Autodesk Fusion 360 part; units mm, degrees
(part 2 of 3)
  spline S19 degree 5 poles (-84.2227, 13.9647) (-84.2245, 13.9707) (-84.2281, 13.9827) (-84.2336, 14.0007) (-84.2409, 14.0246) (-84.2503, 14.0545) (-84.2597, 14.0843) (-84.2693, 14.114) (-84.279, 14.1436) (-84.2888, 14.1731) (-84.2987, 14.2026) (-84.3088, 14.2319) (-84.3189, 14.2612) (-84.3292, 14.2903) (-84.3396, 14.3194) (-84.3502, 14.3484) (-84.3608, 14.3773) (-84.3716, 14.4061) (-84.3825, 14.4348) (-84.3935, 14.4635) (-84.4046, 14.492) (-84.4159, 14.5204) (-84.4273, 14.5488) (-84.4388, 14.577) (-84.4504, 14.6051) (-84.4622, 14.6332) (-84.4741, 14.6611) (-84.4861, 14.6889) (-84.4982, 14.7166) (-84.5105, 14.7442) (-84.5229, 14.7718) (-84.5354, 14.7992) (-84.5481, 14.8264) (-84.5609, 14.8536) (-84.5738, 14.8807) (-84.5869, 14.9076) (-84.6, 14.9345) (-84.6134, 14.9612) (-84.6268, 14.9878) (-84.6404, 15.0143) (-84.6542, 15.0406) (-84.668, 15.0668) (-84.6821, 15.0929) (-84.6962, 15.1189) (-84.7105, 15.1447) (-84.725, 15.1704) (-84.7396, 15.196) (-84.7543, 15.2214) (-84.7692, 15.2467) (-84.7842, 15.2719) (-84.7994, 15.2969) (-84.8148, 15.3217) (-84.8303, 15.3464) (-84.846, 15.3709) (-84.8619, 15.3952) (-84.878, 15.4194) (-84.8941, 15.4435) (-84.9105, 15.4674) (-84.927, 15.4911) (-84.9436, 15.5146) (-84.9605, 15.5379) (-84.9777, 15.561) (-84.9951, 15.5838) (-85.0128, 15.6063) (-85.0307, 15.6286) (-85.0488, 15.6506) (-85.067, 15.6726) (-85.0853, 15.6944) (-85.1038, 15.716) (-85.1226, 15.7372) (-85.142, 15.7579) (-85.1581, 15.7737) (-85.1706, 15.7852) (-85.1791, 15.7926) (-85.1834, 15.7963) knots -1 -1 -1 -1 -1 -1 -0.98571429 -0.97142857 -0.95714286 -0.94285714 -0.92857143 -0.91428571 -0.9 -0.88571429 -0.87142857 -0.85714286 -0.84285714 -0.82857143 -0.81428571 -0.8 -0.78571429 -0.77142857 -0.75714286 -0.74285714 -0.72857143 -0.71428571 -0.7 -0.68571429 -0.67142857 -0.65714286 -0.64285714 -0.62857143 -0.61428571 -0.6 -0.58571429 -0.57142857 -0.55714286 -0.54285714 -0.52857143 -0.51428571 -0.5 -0.48571429 -0.47142857 -0.45714286 -0.44285714 -0.42857143 -0.41428571 -0.4 -0.38571429 -0.37142857 -0.35714286 -0.34285714 -0.32857143 -0.31428571 -0.3 -0.28571429 -0.27142857 -0.25714286 -0.24285714 -0.22857143 -0.21428571 -0.2 -0.18571429 -0.17142857 -0.15714286 -0.14285714 -0.12857143 -0.11428571 -0.1 -0.08571429 -0.07142857 -0.05714286 -0.04285714 -0.02857143 -0.01428571 0 0 0 0 0 0
  line L19 (-85.1834, 15.7963) -> (-85.554, 16.1126)
  arc A39 (-85.5658, 16.2528) -> (-85.554, 16.1126) centre (-85.4891, 16.1886) ccw
  arc A40 (-85.5658, 16.2528) -> (-84.943, 17.0645) centre (-94.8448, 24.0176) ccw
  arc A41 (-84.8044, 17.0894) -> (-84.943, 17.0645) centre (-84.8611, 17.0071) ccw
  line L20 (-84.8044, 17.0894) -> (-84.4031, 16.8133)
  spline S20 degree 5 poles (-84.4031, 16.8133) (-84.3984, 16.8101) (-84.389, 16.8038) (-84.3747, 16.7947) (-84.3552, 16.7833) (-84.3302, 16.7699) (-84.3049, 16.7572) (-84.2792, 16.7449) (-84.2534, 16.7328) (-84.2275, 16.7209) (-84.2015, 16.7092) (-84.1753, 16.6977) (-84.149, 16.6864) (-84.1225, 16.6755) (-84.0958, 16.6649) (-84.0689, 16.6546) (-84.0418, 16.6446) (-84.0147, 16.6348) (-83.9874, 16.6252) (-83.96, 16.6158) (-83.9324, 16.6066) (-83.9048, 16.5975) (-83.8771, 16.5887) (-83.8492, 16.5801) (-83.8213, 16.5717) (-83.7932, 16.5634) (-83.765, 16.5554) (-83.7367, 16.5476) (-83.7083, 16.5399) (-83.6798, 16.5325) (-83.6513, 16.5252) (-83.6226, 16.518) (-83.5939, 16.5111) (-83.565, 16.5043) (-83.5361, 16.4977) (-83.5071, 16.4912) (-83.478, 16.4849) (-83.4488, 16.4788) (-83.4196, 16.4729) (-83.3903, 16.4671) (-83.3608, 16.4614) (-83.3314, 16.456) (-83.3018, 16.4506) (-83.2722, 16.4455) (-83.2425, 16.4405) (-83.2127, 16.4356) (-83.1828, 16.4309) (-83.1529, 16.4263) (-83.1229, 16.4219) (-83.0929, 16.4177) (-83.0627, 16.4136) (-83.0326, 16.4096) (-83.0023, 16.4058) (-82.972, 16.4021) (-82.9416, 16.3986) (-82.9112, 16.3952) (-82.8807, 16.392) (-82.8501, 16.3889) (-82.8195, 16.386) (-82.7888, 16.3832) (-82.7581, 16.3805) (-82.7273, 16.378) (-82.6965, 16.3756) (-82.6656, 16.3734) (-82.6346, 16.3712) (-82.6036, 16.3693) (-82.5726, 16.3674) (-82.5415, 16.3657) (-82.5103, 16.3642) (-82.4791, 16.3628) (-82.4478, 16.3615) (-82.4228, 16.3606) (-82.404, 16.3599) (-82.3914, 16.3595) (-82.3851, 16.3593) knots 0 0 0 0 0 0 0.01428571 0.02857143 0.04285714 0.05714286 0.07142857 0.08571429 0.1 0.11428571 0.12857143 0.14285714 0.15714286 0.17142857 0.18571429 0.2 0.21428571 0.22857143 0.24285714 0.25714286 0.27142857 0.28571429 0.3 0.31428571 0.32857143 0.34285714 0.35714286 0.37142857 0.38571429 0.4 0.41428571 0.42857143 0.44285714 0.45714286 0.47142857 0.48571429 0.5 0.51428571 0.52857143 0.54285714 0.55714286 0.57142857 0.58571429 0.6 0.61428571 0.62857143 0.64285714 0.65714286 0.67142857 0.68571429 0.7 0.71428571 0.72857143 0.74285714 0.75714286 0.77142857 0.78571429 0.8 0.81428571 0.82857143 0.84285714 0.85714286 0.87142857 0.88571429 0.9 0.91428571 0.92857143 0.94285714 0.95714286 0.97142857 0.98571429 1 1 1 1 1 1
  arc A42 (-82.3851, 16.3593) -> (-81.9827, 17.0564) centre (-94.8448, 24.0176) ccw
  spline S21 degree 5 poles (-81.9827, 17.0564) (-81.986, 17.0617) (-81.9926, 17.0724) (-82.0026, 17.0884) (-82.0159, 17.1096) (-82.0326, 17.136) (-82.0495, 17.1624) (-82.0664, 17.1886) (-82.0834, 17.2147) (-82.1005, 17.2406) (-82.1178, 17.2665) (-82.1351, 17.2923) (-82.1524, 17.3179) (-82.1699, 17.3434) (-82.1875, 17.3688) (-82.2052, 17.3941) (-82.223, 17.4193) (-82.2408, 17.4443) (-82.2588, 17.4692) (-82.2768, 17.494) (-82.295, 17.5187) (-82.3132, 17.5432) (-82.3315, 17.5676) (-82.3499, 17.5919) (-82.3685, 17.6161) (-82.3871, 17.6401) (-82.4058, 17.664) (-82.4246, 17.6878) (-82.4435, 17.7114) (-82.4625, 17.7349) (-82.4816, 17.7583) (-82.5008, 17.7815) (-82.5201, 17.8046) (-82.5395, 17.8275) (-82.559, 17.8503) (-82.5785, 17.873) (-82.5982, 17.8955) (-82.618, 17.9178) (-82.6379, 17.9401) (-82.6579, 17.9621) (-82.678, 17.984) (-82.6982, 18.0058) (-82.7185, 18.0273) (-82.7389, 18.0487) (-82.7594, 18.07) (-82.78, 18.0911) (-82.8007, 18.112) (-82.8215, 18.1328) (-82.8424, 18.1533) (-82.8635, 18.1737) (-82.8846, 18.194) (-82.9059, 18.214) (-82.9273, 18.2338) (-82.9488, 18.2534) (-82.9704, 18.2728) (-82.9922, 18.292) (-83.014, 18.311) (-83.036, 18.3299) (-83.0581, 18.3485) (-83.0803, 18.3669) (-83.1026, 18.3851) (-83.1252, 18.4029) (-83.1479, 18.4204) (-83.1708, 18.4376) (-83.1939, 18.4545) (-83.217, 18.4711) (-83.2403, 18.4876) (-83.2636, 18.5039) (-83.2871, 18.52) (-83.3108, 18.5356) (-83.3349, 18.5505) (-83.3545, 18.5617) (-83.3695, 18.5696) (-83.3797, 18.5746) (-83.3848, 18.577) knots -1 -1 -1 -1 -1 -1 -0.98571429 -0.97142857 -0.95714286 -0.94285714 -0.92857143 -0.91428571 -0.9 -0.88571429 -0.87142857 -0.85714286 -0.84285714 -0.82857143 -0.81428571 -0.8 -0.78571429 -0.77142857 -0.75714286 -0.74285714 -0.72857143 -0.71428571 -0.7 -0.68571429 -0.67142857 -0.65714286 -0.64285714 -0.62857143 -0.61428571 -0.6 -0.58571429 -0.57142857 -0.55714286 -0.54285714 -0.52857143 -0.51428571 -0.5 -0.48571429 -0.47142857 -0.45714286 -0.44285714 -0.42857143 -0.41428571 -0.4 -0.38571429 -0.37142857 -0.35714286 -0.34285714 -0.32857143 -0.31428571 -0.3 -0.28571429 -0.27142857 -0.25714286 -0.24285714 -0.22857143 -0.21428571 -0.2 -0.18571429 -0.17142857 -0.15714286 -0.14285714 -0.12857143 -0.11428571 -0.1 -0.08571429 -0.07142857 -0.05714286 -0.04285714 -0.02857143 -0.01428571 0 0 0 0 0 0
  line L21 (-83.3848, 18.577) -> (-83.8246, 18.7865)
  arc A43 (-83.8723, 18.9189) -> (-83.8246, 18.7865) centre (-83.7816, 18.8768) ccw
  arc A44 (-83.8723, 18.9189) -> (-83.4808, 19.8642) centre (-94.8448, 24.0176) ccw
  arc A45 (-83.3534, 19.9241) -> (-83.4808, 19.8642) centre (-83.3868, 19.8299) ccw
  line L22 (-83.3534, 19.9241) -> (-82.8942, 19.7613)
  spline S22 degree 5 poles (-82.8942, 19.7613) (-82.8889, 19.7594) (-82.8782, 19.7557) (-82.862, 19.7507) (-82.8402, 19.7447) (-82.8127, 19.7382) (-82.7849, 19.7325) (-82.7569, 19.7273) (-82.7289, 19.7223) (-82.7008, 19.7175) (-82.6726, 19.7129) (-82.6444, 19.7085) (-82.616, 19.7045) (-82.5876, 19.7008) (-82.559, 19.6975) (-82.5304, 19.6945) (-82.5017, 19.6918) (-82.4729, 19.6894) (-82.444, 19.6872) (-82.4151, 19.6852) (-82.3862, 19.6834) (-82.3571, 19.6818) (-82.3281, 19.6805) (-82.2989, 19.6793) (-82.2697, 19.6785) (-82.2405, 19.6778) (-82.2112, 19.6774) (-82.1818, 19.6771) (-82.1524, 19.6771) (-82.123, 19.6772) (-82.0935, 19.6775) (-82.064, 19.6781) (-82.0344, 19.6788) (-82.0048, 19.6797) (-81.9751, 19.6808) (-81.9455, 19.6821) (-81.9157, 19.6835) (-81.886, 19.6852) (-81.8562, 19.687) (-81.8263, 19.689) (-81.7965, 19.6912) (-81.7666, 19.6935) (-81.7366, 19.696) (-81.7067, 19.6987) (-81.6767, 19.7015) (-81.6467, 19.7046) (-81.6166, 19.7077) (-81.5865, 19.7111) (-81.5564, 19.7146) (-81.5263, 19.7183) (-81.4961, 19.7221) (-81.466, 19.7261) (-81.4358, 19.7302) (-81.4055, 19.7345) (-81.3753, 19.739) (-81.345, 19.7436) (-81.3147, 19.7484) (-81.2844, 19.7533) (-81.2541, 19.7584) (-81.2237, 19.7636) (-81.1933, 19.769) (-81.1629, 19.7745) (-81.1325, 19.7802) (-81.1021, 19.786) (-81.0717, 19.792) (-81.0412, 19.7981) (-81.0107, 19.8044) (-80.9802, 19.8108) (-80.9497, 19.8174) (-80.9192, 19.8241) (-80.8887, 19.8309) (-80.8643, 19.8365) (-80.8459, 19.8408) (-80.8337, 19.8436) (-80.8276, 19.8451) knots 0 0 0 0 0 0 0.01428571 0.02857143 0.04285714 0.05714286 0.07142857 0.08571429 0.1 0.11428571 0.12857143 0.14285714 0.15714286 0.17142857 0.18571429 0.2 0.21428571 0.22857143 0.24285714 0.25714286 0.27142857 0.28571429 0.3 0.31428571 0.32857143 0.34285714 0.35714286 0.37142857 0.38571429 0.4 0.41428571 0.42857143 0.44285714 0.45714286 0.47142857 0.48571429 0.5 0.51428571 0.52857143 0.54285714 0.55714286 0.57142857 0.58571429 0.6 0.61428571 0.62857143 0.64285714 0.65714286 0.67142857 0.68571429 0.7 0.71428571 0.72857143 0.74285714 0.75714286 0.77142857 0.78571429 0.8 0.81428571 0.82857143 0.84285714 0.85714286 0.87142857 0.88571429 0.9 0.91428571 0.92857143 0.94285714 0.95714286 0.97142857 0.98571429 1 1 1 1 1 1
  arc A46 (-80.8276, 19.8451) -> (-80.6193, 20.6225) centre (-94.8448, 24.0176) ccw
  spline S23 degree 5 poles (-80.6193, 20.6225) (-80.6238, 20.6268) (-80.633, 20.6354) (-80.6467, 20.6483) (-80.6651, 20.6654) (-80.6881, 20.6865) (-80.7112, 20.7076) (-80.7343, 20.7285) (-80.7575, 20.7493) (-80.7808, 20.77) (-80.8041, 20.7905) (-80.8275, 20.8109) (-80.8509, 20.8312) (-80.8744, 20.8513) (-80.898, 20.8713) (-80.9216, 20.8911) (-80.9453, 20.9108) (-80.969, 20.9304) (-80.9928, 20.9498) (-81.0166, 20.9691) (-81.0405, 20.9882) (-81.0645, 21.0072) (-81.0885, 21.0261) (-81.1126, 21.0448) (-81.1368, 21.0633) (-81.161, 21.0817) (-81.1852, 21.1) (-81.2095, 21.118) (-81.2339, 21.136) (-81.2583, 21.1538) (-81.2828, 21.1714) (-81.3074, 21.1889) (-81.332, 21.2062) (-81.3567, 21.2233) (-81.3814, 21.2403) (-81.4062, 21.2571) (-81.431, 21.2737) (-81.4559, 21.2902) (-81.4809, 21.3065) (-81.5059, 21.3226) (-81.5309, 21.3386) (-81.5561, 21.3544) (-81.5813, 21.37) (-81.6065, 21.3854) (-81.6318, 21.4006) (-81.6572, 21.4156) (-81.6826, 21.4305) (-81.7081, 21.4451) (-81.7336, 21.4596) (-81.7592, 21.4738) (-81.7849, 21.4879) (-81.8106, 21.5017) (-81.8364, 21.5153) (-81.8623, 21.5287) (-81.8882, 21.5418) (-81.9142, 21.5548) (-81.9402, 21.5675) (-81.9663, 21.58) (-81.9924, 21.5923) (-82.0186, 21.6044) (-82.0449, 21.6161) (-82.0713, 21.6275) (-82.0978, 21.6385) (-82.1244, 21.6492) (-82.151, 21.6595) (-82.1777, 21.6696) (-82.2044, 21.6795) (-82.2312, 21.6892) (-82.258, 21.6987) (-82.285, 21.7076) (-82.3121, 21.7158) (-82.3339, 21.7215) (-82.3505, 21.7252) (-82.3616, 21.7274) (-82.3672, 21.7284) knots -1 -1 -1 -1 -1 -1 -0.98571429 -0.97142857 -0.95714286 -0.94285714 -0.92857143 -0.91428571 -0.9 -0.88571429 -0.87142857 -0.85714286 -0.84285714 -0.82857143 -0.81428571 -0.8 -0.78571429 -0.77142857 -0.75714286 -0.74285714 -0.72857143 -0.71428571 -0.7 -0.68571429 -0.67142857 -0.65714286 -0.64285714 -0.62857143 -0.61428571 -0.6 -0.58571429 -0.57142857 -0.55714286 -0.54285714 -0.52857143 -0.51428571 -0.5 -0.48571429 -0.47142857 -0.45714286 -0.44285714 -0.42857143 -0.41428571 -0.4 -0.38571429 -0.37142857 -0.35714286 -0.34285714 -0.32857143 -0.31428571 -0.3 -0.28571429 -0.27142857 -0.25714286 -0.24285714 -0.22857143 -0.21428571 -0.2 -0.18571429 -0.17142857 -0.15714286 -0.14285714 -0.12857143 -0.11428571 -0.1 -0.08571429 -0.07142857 -0.05714286 -0.04285714 -0.02857143 -0.01428571 0 0 0 0 0 0
  line L23 (-82.3672, 21.7284) -> (-82.8462, 21.817)
  arc A47 (-82.9266, 21.9326) -> (-82.8462, 21.817) centre (-82.8281, 21.9153) ccw
  arc A48 (-82.9266, 21.9326) -> (-82.793, 22.947) centre (-94.8448, 24.0176) ccw
  arc A49 (-82.6855, 23.0378) -> (-82.793, 22.947) centre (-82.6934, 22.9381) ccw
  line L24 (-82.6855, 23.0378) -> (-82.1998, 22.9993)
  spline S24 degree 5 poles (-82.1998, 22.9993) (-82.1942, 22.9989) (-82.1829, 22.9981) (-82.166, 22.9974) (-82.1434, 22.9973) (-82.1151, 22.9982) (-82.0867, 22.9998) (-82.0584, 23.002) (-82.03, 23.0045) (-82.0016, 23.0071) (-81.9732, 23.01) (-81.9448, 23.0131) (-81.9164, 23.0165) (-81.888, 23.0203) (-81.8595, 23.0244) (-81.8311, 23.029) (-81.8027, 23.0338) (-81.7742, 23.0389) (-81.7458, 23.0443) (-81.7173, 23.0498) (-81.6889, 23.0556) (-81.6605, 23.0616) (-81.632, 23.0678) (-81.6036, 23.0743) (-81.5752, 23.081) (-81.5467, 23.0879) (-81.5183, 23.0951) (-81.4899, 23.1024) (-81.4615, 23.11) (-81.4331, 23.1177) (-81.4047, 23.1257) (-81.3763, 23.1338) (-81.3479, 23.1422) (-81.3196, 23.1507) (-81.2912, 23.1595) (-81.2629, 23.1684) (-81.2345, 23.1775) (-81.2062, 23.1868) (-81.1779, 23.1962) (-81.1496, 23.2059) (-81.1213, 23.2157) (-81.093, 23.2257) (-81.0648, 23.2359) (-81.0365, 23.2462) (-81.0083, 23.2568) (-80.9801, 23.2674) (-80.9519, 23.2783) (-80.9237, 23.2893) (-80.8955, 23.3005) (-80.8674, 23.3118) (-80.8392, 23.3233) (-80.8111, 23.335) (-80.783, 23.3468) (-80.7549, 23.3588) (-80.7268, 23.3709) (-80.6988, 23.3832) (-80.6708, 23.3957) (-80.6428, 23.4083) (-80.6148, 23.421) (-80.5868, 23.4339) (-80.5589, 23.447) (-80.5309, 23.4602) (-80.503, 23.4736) (-80.4752, 23.4871) (-80.4473, 23.5007) (-80.4195, 23.5145) (-80.3917, 23.5285) (-80.3639, 23.5425) (-80.3361, 23.5568) (-80.3084, 23.5712) (-80.2806, 23.5857) (-80.2585, 23.5974) (-80.2419, 23.6062) (-80.2308, 23.6122) (-80.2253, 23.6152) knots 0 0 0 0 0 0 0.01428571 0.02857143 0.04285714 0.05714286 0.07142857 0.08571429 0.1 0.11428571 0.12857143 0.14285714 0.15714286 0.17142857 0.18571429 0.2 0.21428571 0.22857143 0.24285714 0.25714286 0.27142857 0.28571429 0.3 0.31428571 0.32857143 0.34285714 0.35714286 0.37142857 0.38571429 0.4 0.41428571 0.42857143 0.44285714 0.45714286 0.47142857 0.48571429 0.5 0.51428571 0.52857143 0.54285714 0.55714286 0.57142857 0.58571429 0.6 0.61428571 0.62857143 0.64285714 0.65714286 0.67142857 0.68571429 0.7 0.71428571 0.72857143 0.74285714 0.75714286 0.77142857 0.78571429 0.8 0.81428571 0.82857143 0.84285714 0.85714286 0.87142857 0.88571429 0.9 0.91428571 0.92857143 0.94285714 0.95714286 0.97142857 0.98571429 1 1 1 1 1 1
  arc A50 (-80.2253, 23.6152) -> (-80.2253, 24.42) centre (-94.8448, 24.0176) ccw
  spline S25 degree 5 poles (-80.2253, 24.42) (-80.2308, 24.423) (-80.2419, 24.429) (-80.2585, 24.4378) (-80.2806, 24.4495) (-80.3084, 24.4641) (-80.3361, 24.4784) (-80.3639, 24.4927) (-80.3917, 24.5067) (-80.4195, 24.5207) (-80.4473, 24.5345) (-80.4752, 24.5481) (-80.503, 24.5616) (-80.5309, 24.575) (-80.5589, 24.5882) (-80.5868, 24.6013) (-80.6148, 24.6142) (-80.6428, 24.6269) (-80.6708, 24.6395) (-80.6988, 24.652) (-80.7268, 24.6643) (-80.7549, 24.6764) (-80.783, 24.6884) (-80.8111, 24.7002) (-80.8392, 24.7119) (-80.8674, 24.7234) (-80.8955, 24.7347) (-80.9237, 24.7459) (-80.9519, 24.7569) (-80.9801, 24.7678) (-81.0083, 24.7785) (-81.0365, 24.789) (-81.0648, 24.7993) (-81.093, 24.8095) (-81.1213, 24.8195) (-81.1496, 24.8293) (-81.1779, 24.839) (-81.2062, 24.8484) (-81.2345, 24.8577) (-81.2629, 24.8668) (-81.2912, 24.8757) (-81.3196, 24.8845) (-81.3479, 24.893) (-81.3763, 24.9014) (-81.4047, 24.9095) (-81.4331, 24.9175) (-81.4615, 24.9252) (-81.4899, 24.9328) (-81.5183, 24.9402) (-81.5467, 24.9473) (-81.5752, 24.9542) (-81.6036, 24.9609) (-81.632, 24.9674) (-81.6605, 24.9736) (-81.6889, 24.9796) (-81.7173, 24.9854) (-81.7458, 24.9909) (-81.7742, 24.9963) (-81.8027, 25.0014) (-81.8311, 25.0062) (-81.8595, 25.0108) (-81.888, 25.0149) (-81.9164, 25.0187) (-81.9448, 25.0221) (-81.9732, 25.0252) (-82.0016, 25.0281) (-82.03, 25.0307) (-82.0584, 25.0332) (-82.0867, 25.0354) (-82.1151, 25.0371) (-82.1434, 25.0379) (-82.166, 25.0378) (-82.1829, 25.0371) (-82.1942, 25.0363) (-82.1998, 25.0359) knots -1 -1 -1 -1 -1 -1 -0.98571429 -0.97142857 -0.95714286 -0.94285714 -0.92857143 -0.91428571 -0.9 -0.88571429 -0.87142857 -0.85714286 -0.84285714 -0.82857143 -0.81428571 -0.8 -0.78571429 -0.77142857 -0.75714286 -0.74285714 -0.72857143 -0.71428571 -0.7 -0.68571429 -0.67142857 -0.65714286 -0.64285714 -0.62857143 -0.61428571 -0.6 -0.58571429 -0.57142857 -0.55714286 -0.54285714 -0.52857143 -0.51428571 -0.5 -0.48571429 -0.47142857 -0.45714286 -0.44285714 -0.42857143 -0.41428571 -0.4 -0.38571429 -0.37142857 -0.35714286 -0.34285714 -0.32857143 -0.31428571 -0.3 -0.28571429 -0.27142857 -0.25714286 -0.24285714 -0.22857143 -0.21428571 -0.2 -0.18571429 -0.17142857 -0.15714286 -0.14285714 -0.12857143 -0.11428571 -0.1 -0.08571429 -0.07142857 -0.05714286 -0.04285714 -0.02857143 -0.01428571 0 0 0 0 0 0
  line L25 (-82.1998, 25.0359) -> (-82.6855, 24.9974)
  arc A51 (-82.793, 25.0883) -> (-82.6855, 24.9974) centre (-82.6934, 25.0971) ccw
  arc A52 (-82.793, 25.0883) -> (-82.9266, 26.1027) centre (-94.8448, 24.0176) ccw
  arc A53 (-82.8462, 26.2182) -> (-82.9266, 26.1027) centre (-82.8281, 26.1199) ccw
  line L26 (-82.8462, 26.2182) -> (-82.3672, 26.3068)
  spline S26 degree 5 poles (-82.3672, 26.3068) (-82.3616, 26.3078) (-82.3505, 26.31) (-82.3339, 26.3137) (-82.3121, 26.3194) (-82.285, 26.3276) (-82.258, 26.3365) (-82.2312, 26.346) (-82.2044, 26.3557) (-82.1777, 26.3656) (-82.151, 26.3757) (-82.1244, 26.386) (-82.0978, 26.3967) (-82.0713, 26.4077) (-82.0449, 26.4191) (-82.0186, 26.4309) (-81.9924, 26.4429) (-81.9663, 26.4552) (-81.9402, 26.4677) (-81.9142, 26.4804) (-81.8882, 26.4934) (-81.8623, 26.5065) (-81.8364, 26.5199) (-81.8106, 26.5335) (-81.7849, 26.5473) (-81.7592, 26.5614) (-81.7336, 26.5756) (-81.7081, 26.5901) (-81.6826, 26.6047) (-81.6572, 26.6196) (-81.6318, 26.6346) (-81.6065, 26.6498) (-81.5813, 26.6652) (-81.5561, 26.6808) (-81.5309, 26.6966) (-81.5059, 26.7126) (-81.4809, 26.7287) (-81.4559, 26.745) (-81.431, 26.7615) (-81.4062, 26.7781) (-81.3814, 26.7949) (-81.3567, 26.8119) (-81.332, 26.829) (-81.3074, 26.8464) (-81.2828, 26.8638) (-81.2583, 26.8814) (-81.2339, 26.8992) (-81.2095, 26.9172) (-81.1852, 26.9352) (-81.161, 26.9535) (-81.1368, 26.9719) (-81.1126, 26.9904) (-81.0885, 27.0091) (-81.0645, 27.028) (-81.0405, 27.047) (-81.0166, 27.0661) (-80.9928, 27.0854) (-80.969, 27.1048) (-80.9453, 27.1244) (-80.9216, 27.1441) (-80.898, 27.1639) (-80.8744, 27.1839) (-80.8509, 27.204) (-80.8275, 27.2243) (-80.8041, 27.2447) (-80.7808, 27.2652) (-80.7575, 27.2859) (-80.7343, 27.3067) (-80.7112, 27.3276) (-80.6881, 27.3487) (-80.6651, 27.3699) (-80.6467, 27.3869) (-80.633, 27.3998) (-80.6238, 27.4084) (-80.6193, 27.4127) knots 0 0 0 0 0 0 0.01428571 0.02857143 0.04285714 0.05714286 0.07142857 0.08571429 0.1 0.11428571 0.12857143 0.14285714 0.15714286 0.17142857 0.18571429 0.2 0.21428571 0.22857143 0.24285714 0.25714286 0.27142857 0.28571429 0.3 0.31428571 0.32857143 0.34285714 0.35714286 0.37142857 0.38571429 0.4 0.41428571 0.42857143 0.44285714 0.45714286 0.47142857 0.48571429 0.5 0.51428571 0.52857143 0.54285714 0.55714286 0.57142857 0.58571429 0.6 0.61428571 0.62857143 0.64285714 0.65714286 0.67142857 0.68571429 0.7 0.71428571 0.72857143 0.74285714 0.75714286 0.77142857 0.78571429 0.8 0.81428571 0.82857143 0.84285714 0.85714286 0.87142857 0.88571429 0.9 0.91428571 0.92857143 0.94285714 0.95714286 0.97142857 0.98571429 1 1 1 1 1 1
  arc A54 (-80.6193, 27.4127) -> (-80.8276, 28.1901) centre (-94.8448, 24.0176) ccw
  spline S27 degree 5 poles (-80.8276, 28.1901) (-80.8337, 28.1916) (-80.8459, 28.1944) (-80.8643, 28.1987) (-80.8887, 28.2043) (-80.9192, 28.2111) (-80.9497, 28.2178) (-80.9802, 28.2244) (-81.0107, 28.2308) (-81.0412, 28.2371) (-81.0717, 28.2432) (-81.1021, 28.2492) (-81.1325, 28.255) (-81.1629, 28.2607) (-81.1933, 28.2662) (-81.2237, 28.2716) (-81.2541, 28.2768) (-81.2844, 28.2819) (-81.3147, 28.2868) (-81.345, 28.2916) (-81.3753, 28.2962) (-81.4055, 28.3007) (-81.4358, 28.305) (-81.466, 28.3091) (-81.4961, 28.3131) (-81.5263, 28.3169) (-81.5564, 28.3206) (-81.5865, 28.3241) (-81.6166, 28.3275) (-81.6467, 28.3307) (-81.6767, 28.3337) (-81.7067, 28.3365) (-81.7366, 28.3392) (-81.7666, 28.3417) (-81.7965, 28.3441) (-81.8263, 28.3462) (-81.8562, 28.3482) (-81.886, 28.35) (-81.9157, 28.3517) (-81.9455, 28.3531) (-81.9751, 28.3544) (-82.0048, 28.3555) (-82.0344, 28.3564) (-82.064, 28.3571) (-82.0935, 28.3577) (-82.123, 28.358) (-82.1524, 28.3581) (-82.1818, 28.3581) (-82.2112, 28.3579) (-82.2405, 28.3574) (-82.2697, 28.3567) (-82.2989, 28.3559) (-82.3281, 28.3547) (-82.3571, 28.3534) (-82.3862, 28.3518) (-82.4151, 28.35) (-82.444, 28.348) (-82.4729, 28.3458) (-82.5017, 28.3434) (-82.5304, 28.3407) (-82.559, 28.3377) (-82.5876, 28.3344) (-82.616, 28.3307) (-82.6444, 28.3267) (-82.6726, 28.3223) (-82.7008, 28.3177) (-82.7289, 28.3129) (-82.7569, 28.3079) (-82.7849, 28.3027) (-82.8127, 28.297) (-82.8402, 28.2905) (-82.862, 28.2845) (-82.8782, 28.2795) (-82.8889, 28.2758) (-82.8942, 28.2739) knots -1 -1 -1 -1 -1 -1 -0.98571429 -0.97142857 -0.95714286 -0.94285714 -0.92857143 -0.91428571 -0.9 -0.88571429 -0.87142857 -0.85714286 -0.84285714 -0.82857143 -0.81428571 -0.8 -0.78571429 -0.77142857 -0.75714286 -0.74285714 -0.72857143 -0.71428571 -0.7 -0.68571429 -0.67142857 -0.65714286 -0.64285714 -0.62857143 -0.61428571 -0.6 -0.58571429 -0.57142857 -0.55714286 -0.54285714 -0.52857143 -0.51428571 -0.5 -0.48571429 -0.47142857 -0.45714286 -0.44285714 -0.42857143 -0.41428571 -0.4 -0.38571429 -0.37142857 -0.35714286 -0.34285714 -0.32857143 -0.31428571 -0.3 -0.28571429 -0.27142857 -0.25714286 -0.24285714 -0.22857143 -0.21428571 -0.2 -0.18571429 -0.17142857 -0.15714286 -0.14285714 -0.12857143 -0.11428571 -0.1 -0.08571429 -0.07142857 -0.05714286 -0.04285714 -0.02857143 -0.01428571 0 0 0 0 0 0
  line L27 (-82.8942, 28.2739) -> (-83.3534, 28.1111)
  arc A55 (-83.4808, 28.171) -> (-83.3534, 28.1111) centre (-83.3868, 28.2053) ccw
  arc A56 (-83.4808, 28.171) -> (-83.8723, 29.1163) centre (-94.8448, 24.0176) ccw
  arc A57 (-83.8246, 29.2487) -> (-83.8723, 29.1163) centre (-83.7816, 29.1584) ccw
  line L28 (-83.8246, 29.2487) -> (-83.3848, 29.4582)
  spline S28 degree 5 poles (-83.3848, 29.4582) (-83.3797, 29.4607) (-83.3695, 29.4656) (-83.3545, 29.4735) (-83.3349, 29.4847) (-83.3108, 29.4996) (-83.2871, 29.5152) (-83.2636, 29.5313) (-83.2403, 29.5476) (-83.217, 29.5641) (-83.1939, 29.5807) (-83.1708, 29.5976) (-83.1479, 29.6148) (-83.1252, 29.6323) (-83.1026, 29.6501) (-83.0803, 29.6683) (-83.0581, 29.6867) (-83.036, 29.7053) (-83.014, 29.7242) (-82.9922, 29.7432) (-82.9704, 29.7624) (-82.9488, 29.7818) (-82.9273, 29.8014) (-82.9059, 29.8212) (-82.8846, 29.8412) (-82.8635, 29.8615) (-82.8424, 29.8819) (-82.8215, 29.9025) (-82.8007, 29.9232) (-82.78, 29.9441) (-82.7594, 29.9652) (-82.7389, 29.9865) (-82.7185, 30.0079) (-82.6982, 30.0295) (-82.678, 30.0512) (-82.6579, 30.0731) (-82.6379, 30.0952) (-82.618, 30.1174) (-82.5982, 30.1397) (-82.5785, 30.1622) (-82.559, 30.1849) (-82.5395, 30.2077) (-82.5201, 30.2306) (-82.5008, 30.2537) (-82.4816, 30.2769) (-82.4625, 30.3003) (-82.4435, 30.3238) (-82.4246, 30.3474) (-82.4058, 30.3712) (-82.3871, 30.3951) (-82.3685, 30.4191) (-82.3499, 30.4433) (-82.3315, 30.4676) (-82.3132, 30.492) (-82.295, 30.5165) (-82.2768, 30.5412) (-82.2588, 30.566) (-82.2408, 30.5909) (-82.223, 30.616) (-82.2052, 30.6411) (-82.1875, 30.6664) (-82.1699, 30.6918) (-82.1524, 30.7173) (-82.1351, 30.7429) (-82.1178, 30.7687) (-82.1005, 30.7946) (-82.0834, 30.8205) (-82.0664, 30.8466) (-82.0495, 30.8728) (-82.0326, 30.8992) (-82.0159, 30.9256) (-82.0026, 30.9468) (-81.9926, 30.9628) (-81.986, 30.9735) (-81.9827, 30.9788) knots 0 0 0 0 0 0 0.01428571 0.02857143 0.04285714 0.05714286 0.07142857 0.08571429 0.1 0.11428571 0.12857143 0.14285714 0.15714286 0.17142857 0.18571429 0.2 0.21428571 0.22857143 0.24285714 0.25714286 0.27142857 0.28571429 0.3 0.31428571 0.32857143 0.34285714 0.35714286 0.37142857 0.38571429 0.4 0.41428571 0.42857143 0.44285714 0.45714286 0.47142857 0.48571429 0.5 0.51428571 0.52857143 0.54285714 0.55714286 0.57142857 0.58571429 0.6 0.61428571 0.62857143 0.64285714 0.65714286 0.67142857 0.68571429 0.7 0.71428571 0.72857143 0.74285714 0.75714286 0.77142857 0.78571429 0.8 0.81428571 0.82857143 0.84285714 0.85714286 0.87142857 0.88571429 0.9 0.91428571 0.92857143 0.94285714 0.95714286 0.97142857 0.98571429 1 1 1 1 1 1
  arc A58 (-81.9827, 30.9788) -> (-82.3851, 31.6759) centre (-94.8448, 24.0176) ccw
  spline S29 degree 5 poles (-82.3851, 31.6759) (-82.3914, 31.6757) (-82.404, 31.6753) (-82.4228, 31.6746) (-82.4478, 31.6737) (-82.4791, 31.6724) (-82.5103, 31.671) (-82.5415, 31.6695) (-82.5726, 31.6678) (-82.6036, 31.6659) (-82.6346, 31.664) (-82.6656, 31.6619) (-82.6965, 31.6596) (-82.7273, 31.6572) (-82.7581, 31.6547) (-82.7888, 31.652) (-82.8195, 31.6492) (-82.8501, 31.6463) (-82.8807, 31.6432) (-82.9112, 31.64) (-82.9416, 31.6366) (-82.972, 31.6331) (-83.0023, 31.6294) (-83.0326, 31.6256) (-83.0627, 31.6216) (-83.0929, 31.6175) (-83.1229, 31.6133) (-83.1529, 31.6089) (-83.1828, 31.6043) (-83.2127, 31.5996) (-83.2425, 31.5948) (-83.2722, 31.5897) (-83.3018, 31.5846) (-83.3314, 31.5793) (-83.3608, 31.5738) (-83.3903, 31.5681) (-83.4196, 31.5623) (-83.4488, 31.5564) (-83.478, 31.5503) (-83.5071, 31.544) (-83.5361, 31.5375) (-83.565, 31.5309) (-83.5939, 31.5241) (-83.6226, 31.5172) (-83.6513, 31.51) (-83.6798, 31.5027) (-83.7083, 31.4953) (-83.7367, 31.4876) (-83.765, 31.4798) (-83.7932, 31.4718) (-83.8213, 31.4636) (-83.8492, 31.4551) (-83.8771, 31.4465) (-83.9048, 31.4377) (-83.9324, 31.4287) (-83.96, 31.4194) (-83.9874, 31.41) (-84.0147, 31.4004) (-84.0418, 31.3906) (-84.0689, 31.3806) (-84.0958, 31.3703) (-84.1225, 31.3597) (-84.149, 31.3488) (-84.1753, 31.3375) (-84.2015, 31.326) (-84.2275, 31.3143) (-84.2534, 31.3024) (-84.2792, 31.2903) (-84.3049, 31.278) (-84.3302, 31.2653) (-84.3552, 31.2519) (-84.3747, 31.2405) (-84.389, 31.2314) (-84.3984, 31.2251) (-84.4031, 31.2219) knots -1 -1 -1 -1 -1 -1 -0.98571429 -0.97142857 -0.95714286 -0.94285714 -0.92857143 -0.91428571 -0.9 -0.88571429 -0.87142857 -0.85714286 -0.84285714 -0.82857143 -0.81428571 -0.8 -0.78571429 -0.77142857 -0.75714286 -0.74285714 -0.72857143 -0.71428571 -0.7 -0.68571429 -0.67142857 -0.65714286 -0.64285714 -0.62857143 -0.61428571 -0.6 -0.58571429 -0.57142857 -0.55714286 -0.54285714 -0.52857143 -0.51428571 -0.5 -0.48571429 -0.47142857 -0.45714286 -0.44285714 -0.42857143 -0.41428571 -0.4 -0.38571429 -0.37142857 -0.35714286 -0.34285714 -0.32857143 -0.31428571 -0.3 -0.28571429 -0.27142857 -0.25714286 -0.24285714 -0.22857143 -0.21428571 -0.2 -0.18571429 -0.17142857 -0.15714286 -0.14285714 -0.12857143 -0.11428571 -0.1 -0.08571429 -0.07142857 -0.05714286 -0.04285714 -0.02857143 -0.01428571 0 0 0 0 0 0
  line L29 (-84.4031, 31.2219) -> (-84.8044, 30.9458)
  arc A59 (-84.943, 30.9707) -> (-84.8044, 30.9458) centre (-84.8611, 31.0281) ccw
  arc A60 (-84.943, 30.9707) -> (-85.5658, 31.7824) centre (-94.8448, 24.0176) ccw
  arc A61 (-85.554, 31.9227) -> (-85.5658, 31.7824) centre (-85.4891, 31.8466) ccw
  line L30 (-85.554, 31.9227) -> (-85.1834, 32.2389)
  spline S30 degree 5 poles (-85.1834, 32.2389) (-85.1791, 32.2426) (-85.1706, 32.25) (-85.1581, 32.2615) (-85.142, 32.2774) (-85.1226, 32.298) (-85.1038, 32.3192) (-85.0853, 32.3408) (-85.067, 32.3626) (-85.0488, 32.3846) (-85.0307, 32.4067) (-85.0128, 32.4289) (-84.9951, 32.4514) (-84.9777, 32.4742) (-84.9605, 32.4973) (-84.9436, 32.5206) (-84.927, 32.5441) (-84.9105, 32.5679) (-84.8941, 32.5917) (-84.878, 32.6158) (-84.8619, 32.64) (-84.846, 32.6643) (-84.8303, 32.6888) (-84.8148, 32.7135) (-84.7994, 32.7383) (-84.7842, 32.7633) (-84.7692, 32.7885) (-84.7543, 32.8138) (-84.7396, 32.8392) (-84.725, 32.8648) (-84.7105, 32.8905) (-84.6962, 32.9163) (-84.6821, 32.9423) (-84.668, 32.9684) (-84.6542, 32.9946) (-84.6404, 33.021) (-84.6268, 33.0474) (-84.6134, 33.074) (-84.6, 33.1007) (-84.5869, 33.1276) (-84.5738, 33.1545) (-84.5609, 33.1816) (-84.5481, 33.2088) (-84.5354, 33.2361) (-84.5229, 33.2635) (-84.5105, 33.291) (-84.4982, 33.3186) (-84.4861, 33.3463) (-84.4741, 33.3741) (-84.4622, 33.4021) (-84.4504, 33.4301) (-84.4388, 33.4582) (-84.4273, 33.4865) (-84.4159, 33.5148) (-84.4046, 33.5432) (-84.3935, 33.5717) (-84.3825, 33.6004) (-84.3716, 33.6291) (-84.3608, 33.6579) (-84.3502, 33.6868) (-84.3396, 33.7158) (-84.3292, 33.7449) (-84.3189, 33.774) (-84.3088, 33.8033) (-84.2987, 33.8327) (-84.2888, 33.8621) (-84.279, 33.8916) (-84.2693, 33.9212) (-84.2597, 33.9509) (-84.2503, 33.9807) (-84.2409, 34.0106) (-84.2336, 34.0345) (-84.2281, 34.0525) (-84.2245, 34.0645) (-84.2227, 34.0706) knots 0 0 0 0 0 0 0.01428571 0.02857143 0.04285714 0.05714286 0.07142857 0.08571429 0.1 0.11428571 0.12857143 0.14285714 0.15714286 0.17142857 0.18571429 0.2 0.21428571 0.22857143 0.24285714 0.25714286 0.27142857 0.28571429 0.3 0.31428571 0.32857143 0.34285714 0.35714286 0.37142857 0.38571429 0.4 0.41428571 0.42857143 0.44285714 0.45714286 0.47142857 0.48571429 0.5 0.51428571 0.52857143 0.54285714 0.55714286 0.57142857 0.58571429 0.6 0.61428571 0.62857143 0.64285714 0.65714286 0.67142857 0.68571429 0.7 0.71428571 0.72857143 0.74285714 0.75714286 0.77142857 0.78571429 0.8 0.81428571 0.82857143 0.84285714 0.85714286 0.87142857 0.88571429 0.9 0.91428571 0.92857143 0.94285714 0.95714286 0.97142857 0.98571429 1 1 1 1 1 1
  arc A62 (-84.2227, 34.0706) -> (-84.7918, 34.6397) centre (-94.8448, 24.0176) ccw
  spline S31 degree 5 poles (-84.7918, 34.6397) (-84.7978, 34.6379) (-84.8098, 34.6343) (-84.8278, 34.6288) (-84.8518, 34.6214) (-84.8817, 34.6121) (-84.9114, 34.6026) (-84.9411, 34.5931) (-84.9707, 34.5834) (-85.0003, 34.5736) (-85.0297, 34.5636) (-85.0591, 34.5536) (-85.0883, 34.5434) (-85.1175, 34.5331) (-85.1466, 34.5227) (-85.1756, 34.5122) (-85.2045, 34.5015) (-85.2333, 34.4908) (-85.262, 34.4799) (-85.2906, 34.4689) (-85.3191, 34.4577) (-85.3476, 34.4465) (-85.3759, 34.4351) (-85.4041, 34.4236) (-85.4323, 34.4119) (-85.4603, 34.4002) (-85.4882, 34.3883) (-85.5161, 34.3763) (-85.5438, 34.3641) (-85.5714, 34.3519) (-85.5989, 34.3395) (-85.6263, 34.3269) (-85.6536, 34.3143) (-85.6808, 34.3015) (-85.7078, 34.2886) (-85.7348, 34.2755) (-85.7616, 34.2623) (-85.7883, 34.249) (-85.8149, 34.2355) (-85.8414, 34.2219) (-85.8678, 34.2082) (-85.894, 34.1943) (-85.9201, 34.1803) (-85.946, 34.1661) (-85.9719, 34.1518) (-85.9976, 34.1374) (-86.0231, 34.1228) (-86.0486, 34.108) (-86.0739, 34.0932) (-86.099, 34.0781) (-86.124, 34.0629) (-86.1489, 34.0476) (-86.1735, 34.032) (-86.1981, 34.0163) (-86.2224, 34.0004) (-86.2466, 33.9844) (-86.2706, 33.9682) (-86.2945, 33.9519) (-86.3182, 33.9354) (-86.3418, 33.9187) (-86.3651, 33.9018) (-86.3881, 33.8847) (-86.4109, 33.8672) (-86.4334, 33.8496) (-86.4557, 33.8317) (-86.4778, 33.8136) (-86.4997, 33.7954) (-86.5215, 33.7771) (-86.5431, 33.7586) (-86.5644, 33.7397) (-86.585, 33.7203) (-86.6009, 33.7042) (-86.6123, 33.6917) (-86.6198, 33.6832) (-86.6235, 33.6789) knots -1 -1 -1 -1 -1 -1 -0.98571429 -0.97142857 -0.95714286 -0.94285714 -0.92857143 -0.91428571 -0.9 -0.88571429 -0.87142857 -0.85714286 -0.84285714 -0.82857143 -0.81428571 -0.8 -0.78571429 -0.77142857 -0.75714286 -0.74285714 -0.72857143 -0.71428571 -0.7 -0.68571429 -0.67142857 -0.65714286 -0.64285714 -0.62857143 -0.61428571 -0.6 -0.58571429 -0.57142857 -0.55714286 -0.54285714 -0.52857143 -0.51428571 -0.5 -0.48571429 -0.47142857 -0.45714286 -0.44285714 -0.42857143 -0.41428571 -0.4 -0.38571429 -0.37142857 -0.35714286 -0.34285714 -0.32857143 -0.31428571 -0.3 -0.28571429 -0.27142857 -0.25714286 -0.24285714 -0.22857143 -0.21428571 -0.2 -0.18571429 -0.17142857 -0.15714286 -0.14285714 -0.12857143 -0.11428571 -0.1 -0.08571429 -0.07142857 -0.05714286 -0.04285714 -0.02857143 -0.01428571 0 0 0 0 0 0
  line L31 (-86.6235, 33.6789) -> (-86.9397, 33.3083)
  arc A63 (-87.08, 33.2965) -> (-86.9397, 33.3083) centre (-87.0158, 33.3732) ccw
  arc A64 (-87.08, 33.2965) -> (-87.8917, 33.9194) centre (-94.8448, 24.0176) ccw
  arc A65 (-87.9166, 34.0579) -> (-87.8917, 33.9194) centre (-87.8342, 34.0012) ccw
  line L32 (-87.9166, 34.0579) -> (-87.6404, 34.4593)
  spline S32 degree 5 poles (-87.6404, 34.4593) (-87.6372, 34.464) (-87.6309, 34.4733) (-87.6219, 34.4877) (-87.6104, 34.5072) (-87.597, 34.5321) (-87.5843, 34.5575) (-87.572, 34.5831) (-87.56, 34.6089) (-87.5481, 34.6349) (-87.5363, 34.6609) (-87.5248, 34.687) (-87.5136, 34.7133) (-87.5026, 34.7398) (-87.492, 34.7666) (-87.4818, 34.7935) (-87.4717, 34.8205) (-87.4619, 34.8477) (-87.4523, 34.875) (-87.4429, 34.9024) (-87.4337, 34.9299) (-87.4247, 34.9575) (-87.4158, 34.9853) (-87.4072, 35.0131) (-87.3988, 35.0411) (-87.3906, 35.0692) (-87.3826, 35.0974) (-87.3747, 35.1256) (-87.3671, 35.154) (-87.3596, 35.1825) (-87.3523, 35.2111) (-87.3452, 35.2397) (-87.3382, 35.2685) (-87.3314, 35.2973) (-87.3248, 35.3262) (-87.3184, 35.3552) (-87.3121, 35.3843) (-87.306, 35.4135) (-87.3, 35.4428) (-87.2942, 35.4721) (-87.2886, 35.5015) (-87.2831, 35.531) (-87.2778, 35.5606) (-87.2726, 35.5902) (-87.2676, 35.6199) (-87.2627, 35.6497) (-87.258, 35.6795) (-87.2535, 35.7095) (-87.2491, 35.7394) (-87.2448, 35.7695) (-87.2407, 35.7996) (-87.2368, 35.8298) (-87.233, 35.86) (-87.2293, 35.8904) (-87.2258, 35.9207) (-87.2224, 35.9512) (-87.2192, 35.9817) (-87.2161, 36.0122) (-87.2131, 36.0428) (-87.2103, 36.0735) (-87.2077, 36.1042) (-87.2051, 36.135) (-87.2027, 36.1659) (-87.2005, 36.1968) (-87.1984, 36.2277) (-87.1964, 36.2587) (-87.1946, 36.2898) (-87.1929, 36.3209) (-87.1913, 36.3521) (-87.1899, 36.3833) (-87.1886, 36.4145) (-87.1877, 36.4396) (-87.1871, 36.4584) (-87.1867, 36.4709) (-87.1865, 36.4772) knots 0 0 0 0 0 0 0.01428571 0.02857143 0.04285714 0.05714286 0.07142857 0.08571429 0.1 0.11428571 0.12857143 0.14285714 0.15714286 0.17142857 0.18571429 0.2 0.21428571 0.22857143 0.24285714 0.25714286 0.27142857 0.28571429 0.3 0.31428571 0.32857143 0.34285714 0.35714286 0.37142857 0.38571429 0.4 0.41428571 0.42857143 0.44285714 0.45714286 0.47142857 0.48571429 0.5 0.51428571 0.52857143 0.54285714 0.55714286 0.57142857 0.58571429 0.6 0.61428571 0.62857143 0.64285714 0.65714286 0.67142857 0.68571429 0.7 0.71428571 0.72857143 0.74285714 0.75714286 0.77142857 0.78571429 0.8 0.81428571 0.82857143 0.84285714 0.85714286 0.87142857 0.88571429 0.9 0.91428571 0.92857143 0.94285714 0.95714286 0.97142857 0.98571429 1 1 1 1 1 1
  arc A66 (-87.1865, 36.4772) -> (-87.8835, 36.8797) centre (-94.8448, 24.0176) ccw
  spline S33 degree 5 poles (-87.8835, 36.8797) (-87.8889, 36.8763) (-87.8996, 36.8697) (-87.9155, 36.8598) (-87.9368, 36.8465) (-87.9632, 36.8297) (-87.9895, 36.8129) (-88.0157, 36.7959) (-88.0418, 36.7789) (-88.0678, 36.7618) (-88.0937, 36.7446) (-88.1194, 36.7273) (-88.145, 36.7099) (-88.1706, 36.6924) (-88.196, 36.6748) (-88.2212, 36.6572) (-88.2464, 36.6394) (-88.2714, 36.6215) (-88.2964, 36.6036) (-88.3212, 36.5855) (-88.3458, 36.5674) (-88.3704, 36.5492) (-88.3948, 36.5308) (-88.4191, 36.5124) (-88.4432, 36.4939) (-88.4673, 36.4753) (-88.4912, 36.4566) (-88.5149, 36.4378) (-88.5386, 36.4189) (-88.5621, 36.3999) (-88.5854, 36.3808) (-88.6087, 36.3616) (-88.6317, 36.3423) (-88.6547, 36.3229) (-88.6775, 36.3034) (-88.7001, 36.2838) (-88.7226, 36.2641) (-88.745, 36.2443) (-88.7672, 36.2245) (-88.7893, 36.2045) (-88.8112, 36.1844) (-88.8329, 36.1642) (-88.8545, 36.1439) (-88.8759, 36.1235) (-88.8971, 36.103) (-88.9182, 36.0824) (-88.9391, 36.0617) (-88.9599, 36.0408) (-88.9805, 36.0199) (-89.0009, 35.9989) (-89.0211, 35.9777) (-89.0411, 35.9565) (-89.0609, 35.9351) (-89.0805, 35.9135) (-89.0999, 35.8919) (-89.1192, 35.8702) (-89.1382, 35.8483) (-89.157, 35.8263) (-89.1757, 35.8043) (-89.1941, 35.7821) (-89.2122, 35.7597) (-89.2301, 35.7372) (-89.2476, 35.7145) (-89.2647, 35.6916) (-89.2816, 35.6685) (-89.2983, 35.6453) (-89.3148, 35.6221) (-89.3311, 35.5987) (-89.3472, 35.5753) (-89.3628, 35.5516) (-89.3777, 35.5275) (-89.3889, 35.5078) (-89.3967, 35.4928) (-89.4017, 35.4827) (-89.4041, 35.4776) knots -1 -1 -1 -1 -1 -1 -0.98571429 -0.97142857 -0.95714286 -0.94285714 -0.92857143 -0.91428571 -0.9 -0.88571429 -0.87142857 -0.85714286 -0.84285714 -0.82857143 -0.81428571 -0.8 -0.78571429 -0.77142857 -0.75714286 -0.74285714 -0.72857143 -0.71428571 -0.7 -0.68571429 -0.67142857 -0.65714286 -0.64285714 -0.62857143 -0.61428571 -0.6 -0.58571429 -0.57142857 -0.55714286 -0.54285714 -0.52857143 -0.51428571 -0.5 -0.48571429 -0.47142857 -0.45714286 -0.44285714 -0.42857143 -0.41428571 -0.4 -0.38571429 -0.37142857 -0.35714286 -0.34285714 -0.32857143 -0.31428571 -0.3 -0.28571429 -0.27142857 -0.25714286 -0.24285714 -0.22857143 -0.21428571 -0.2 -0.18571429 -0.17142857 -0.15714286 -0.14285714 -0.12857143 -0.11428571 -0.1 -0.08571429 -0.07142857 -0.05714286 -0.04285714 -0.02857143 -0.01428571 0 0 0 0 0 0
  line L33 (-89.4041, 35.4776) -> (-89.6137, 35.0377)
  arc A67 (-89.7461, 34.99) -> (-89.6137, 35.0377) centre (-89.704, 35.0807) ccw
  arc A68 (-89.7461, 34.99) -> (-90.6914, 35.3816) centre (-94.8448, 24.0176) ccw
  arc A69 (-90.7513, 35.5089) -> (-90.6914, 35.3816) centre (-90.657, 35.4755) ccw
  line L34 (-90.7513, 35.5089) -> (-90.5884, 35.9681)
  spline S34 degree 5 poles (-90.5884, 35.9681) (-90.5865, 35.9734) (-90.5829, 35.9841) (-90.5778, 36.0003) (-90.5718, 36.0221) (-90.5654, 36.0497) (-90.5596, 36.0775) (-90.5544, 36.1054) (-90.5494, 36.1335) (-90.5447, 36.1616) (-90.5401, 36.1898) (-90.5357, 36.218) (-90.5316, 36.2463) (-90.5279, 36.2748) (-90.5246, 36.3033) (-90.5216, 36.332) (-90.519, 36.3607) (-90.5165, 36.3895) (-90.5143, 36.4183) (-90.5123, 36.4472) (-90.5105, 36.4762) (-90.509, 36.5052) (-90.5076, 36.5343) (-90.5065, 36.5634) (-90.5056, 36.5926) (-90.5049, 36.6219) (-90.5045, 36.6512) (-90.5043, 36.6805) (-90.5042, 36.7099) (-90.5044, 36.7394) (-90.5047, 36.7689) (-90.5052, 36.7984) (-90.5059, 36.8279) (-90.5068, 36.8576) (-90.5079, 36.8872) (-90.5092, 36.9169) (-90.5107, 36.9466) (-90.5123, 36.9764) (-90.5141, 37.0062) (-90.5161, 37.036) (-90.5183, 37.0659) (-90.5206, 37.0958) (-90.5232, 37.1257) (-90.5258, 37.1557) (-90.5287, 37.1857) (-90.5317, 37.2157) (-90.5349, 37.2457) (-90.5382, 37.2758) (-90.5417, 37.3059) (-90.5454, 37.3361) (-90.5492, 37.3662) (-90.5532, 37.3964) (-90.5574, 37.4266) (-90.5617, 37.4568) (-90.5661, 37.4871) (-90.5708, 37.5174) (-90.5755, 37.5477) (-90.5805, 37.578) (-90.5855, 37.6083) (-90.5908, 37.6387) (-90.5961, 37.669) (-90.6017, 37.6994) (-90.6073, 37.7298) (-90.6132, 37.7603) (-90.6191, 37.7907) (-90.6253, 37.8212) (-90.6315, 37.8516) (-90.638, 37.8821) (-90.6445, 37.9126) (-90.6512, 37.9431) (-90.6581, 37.9737) (-90.6637, 37.9981) (-90.6679, 38.0164) (-90.6708, 38.0286) (-90.6722, 38.0348) knots 0 0 0 0 0 0 0.01428571 0.02857143 0.04285714 0.05714286 0.07142857 0.08571429 0.1 0.11428571 0.12857143 0.14285714 0.15714286 0.17142857 0.18571429 0.2 0.21428571 0.22857143 0.24285714 0.25714286 0.27142857 0.28571429 0.3 0.31428571 0.32857143 0.34285714 0.35714286 0.37142857 0.38571429 0.4 0.41428571 0.42857143 0.44285714 0.45714286 0.47142857 0.48571429 0.5 0.51428571 0.52857143 0.54285714 0.55714286 0.57142857 0.58571429 0.6 0.61428571 0.62857143 0.64285714 0.65714286 0.67142857 0.68571429 0.7 0.71428571 0.72857143 0.74285714 0.75714286 0.77142857 0.78571429 0.8 0.81428571 0.82857143 0.84285714 0.85714286 0.87142857 0.88571429 0.9 0.91428571 0.92857143 0.94285714 0.95714286 0.97142857 0.98571429 1 1 1 1 1 1
  arc A70 (-90.6722, 38.0348) -> (-91.4497, 38.2431) centre (-94.8448, 24.0176) ccw
  spline S35 degree 5 poles (-91.4497, 38.2431) (-91.454, 38.2385) (-91.4626, 38.2294) (-91.4754, 38.2156) (-91.4925, 38.1972) (-91.5137, 38.1742) (-91.5348, 38.1512) (-91.5557, 38.128) (-91.5765, 38.1048) (-91.5972, 38.0816) (-91.6177, 38.0583) (-91.6381, 38.0349) (-91.6583, 38.0114) (-91.6785, 37.9879) (-91.6984, 37.9644) (-91.7183, 37.9408) (-91.738, 37.9171) (-91.7576, 37.8934) (-91.777, 37.8696) (-91.7963, 37.8457) (-91.8154, 37.8218) (-91.8344, 37.7979) (-91.8532, 37.7738) (-91.8719, 37.7497) (-91.8905, 37.7256) (-91.9089, 37.7014) (-91.9271, 37.6771) (-91.9452, 37.6528) (-91.9631, 37.6284) (-91.9809, 37.604) (-91.9985, 37.5795) (-92.016, 37.555) (-92.0333, 37.5304) (-92.0504, 37.5057) (-92.0674, 37.481) (-92.0842, 37.4562) (-92.1009, 37.4314) (-92.1174, 37.4065) (-92.1337, 37.3815) (-92.1498, 37.3565) (-92.1657, 37.3314) (-92.1815, 37.3063) (-92.1971, 37.2811) (-92.2125, 37.2558) (-92.2277, 37.2305) (-92.2428, 37.2052) (-92.2576, 37.1797) (-92.2723, 37.1543) (-92.2867, 37.1287) (-92.301, 37.1031) (-92.315, 37.0775) (-92.3289, 37.0517) (-92.3425, 37.0259) (-92.3558, 37.0001) (-92.369, 36.9742) (-92.3819, 36.9482) (-92.3946, 36.9222) (-92.4072, 36.8961) (-92.4195, 36.8699) (-92.4315, 36.8437) (-92.4432, 36.8174) (-92.4546, 36.791) (-92.4657, 36.7646) (-92.4763, 36.738) (-92.4866, 36.7113) (-92.4967, 36.6847) (-92.5067, 36.6579) (-92.5164, 36.6311) (-92.5258, 36.6043) (-92.5348, 36.5774) (-92.543, 36.5503) (-92.5487, 36.5284) (-92.5524, 36.5119) (-92.5545, 36.5008) (-92.5556, 36.4952) knots -1 -1 -1 -1 -1 -1 -0.98571429 -0.97142857 -0.95714286 -0.94285714 -0.92857143 -0.91428571 -0.9 -0.88571429 -0.87142857 -0.85714286 -0.84285714 -0.82857143 -0.81428571 -0.8 -0.78571429 -0.77142857 -0.75714286 -0.74285714 -0.72857143 -0.71428571 -0.7 -0.68571429 -0.67142857 -0.65714286 -0.64285714 -0.62857143 -0.61428571 -0.6 -0.58571429 -0.57142857 -0.55714286 -0.54285714 -0.52857143 -0.51428571 -0.5 -0.48571429 -0.47142857 -0.45714286 -0.44285714 -0.42857143 -0.41428571 -0.4 -0.38571429 -0.37142857 -0.35714286 -0.34285714 -0.32857143 -0.31428571 -0.3 -0.28571429 -0.27142857 -0.25714286 -0.24285714 -0.22857143 -0.21428571 -0.2 -0.18571429 -0.17142857 -0.15714286 -0.14285714 -0.12857143 -0.11428571 -0.1 -0.08571429 -0.07142857 -0.05714286 -0.04285714 -0.02857143 -0.01428571 0 0 0 0 0 0
  line L35 (-92.5556, 36.4952) -> (-92.6441, 36.0161)
  arc A71 (-92.7597, 35.9358) -> (-92.6441, 36.0161) centre (-92.7425, 36.0343) ccw
  arc A72 (-92.7597, 35.9358) -> (-93.7741, 36.0693) centre (-94.8448, 24.0176) ccw
  arc A73 (-93.8649, 36.1768) -> (-93.7741, 36.0693) centre (-93.7653, 36.1689) ccw
  line L36 (-93.8649, 36.1768) -> (-93.8265, 36.6625)
  spline S36 degree 5 poles (-93.8265, 36.6625) (-93.826, 36.6682) (-93.8253, 36.6794) (-93.8246, 36.6964) (-93.8244, 36.719) (-93.8253, 36.7473) (-93.827, 36.7756) (-93.8292, 36.804) (-93.8316, 36.8324) (-93.8343, 36.8607) (-93.8371, 36.8891) (-93.8402, 36.9176) (-93.8436, 36.946) (-93.8474, 36.9744) (-93.8516, 37.0028) (-93.8561, 37.0313) (-93.861, 37.0597) (-93.8661, 37.0881) (-93.8714, 37.1166) (-93.877, 37.145) (-93.8827, 37.1735) (-93.8887, 37.2019) (-93.895, 37.2303) (-93.9014, 37.2588) (-93.9081, 37.2872) (-93.915, 37.3156) (-93.9222, 37.344) (-93.9296, 37.3725) (-93.9371, 37.4009) (-93.9449, 37.4293) (-93.9528, 37.4577) (-93.961, 37.486) (-93.9693, 37.5144) (-93.9779, 37.5428) (-93.9866, 37.5711) (-93.9955, 37.5995) (-94.0046, 37.6278) (-94.0139, 37.6561) (-94.0234, 37.6845) (-94.033, 37.7128) (-94.0429, 37.741) (-94.0529, 37.7693) (-94.063, 37.7976) (-94.0734, 37.8258) (-94.0839, 37.8541) (-94.0946, 37.8823) (-94.1054, 37.9105) (-94.1165, 37.9387) (-94.1276, 37.9668) (-94.139, 37.995) (-94.1505, 38.0231) (-94.1621, 38.0513) (-94.174, 38.0794) (-94.1859, 38.1074) (-94.1981, 38.1355) (-94.2104, 38.1636) (-94.2228, 38.1916) (-94.2354, 38.2196) (-94.2482, 38.2476) (-94.2611, 38.2755) (-94.2742, 38.3035) (-94.2874, 38.3314) (-94.3007, 38.3593) (-94.3142, 38.3872) (-94.3279, 38.4151) (-94.3417, 38.4429) (-94.3556, 38.4707) (-94.3697, 38.4985) (-94.3839, 38.5263) (-94.3983, 38.554) (-94.4128, 38.5817) (-94.4245, 38.6039) (-94.4334, 38.6205) (-94.4393, 38.6315) (-94.4423, 38.6371) knots 0 0 0 0 0 0 0.01428571 0.02857143 0.04285714 0.05714286 0.07142857 0.08571429 0.1 0.11428571 0.12857143 0.14285714 0.15714286 0.17142857 0.18571429 0.2 0.21428571 0.22857143 0.24285714 0.25714286 0.27142857 0.28571429 0.3 0.31428571 0.32857143 0.34285714 0.35714286 0.37142857 0.38571429 0.4 0.41428571 0.42857143 0.44285714 0.45714286 0.47142857 0.48571429 0.5 0.51428571 0.52857143 0.54285714 0.55714286 0.57142857 0.58571429 0.6 0.61428571 0.62857143 0.64285714 0.65714286 0.67142857 0.68571429 0.7 0.71428571 0.72857143 0.74285714 0.75714286 0.77142857 0.78571429 0.8 0.81428571 0.82857143 0.84285714 0.85714286 0.87142857 0.88571429 0.9 0.91428571 0.92857143 0.94285714 0.95714286 0.97142857 0.98571429 1 1 1 1 1 1
  arc A74 (-94.4423, 38.6371) -> (-95.2472, 38.6371) centre (-94.8448, 24.0176) ccw
  spline S37 degree 5 poles (-95.2472, 38.6371) (-95.2502, 38.6315) (-95.2561, 38.6205) (-95.265, 38.6039) (-95.2767, 38.5817) (-95.2912, 38.554) (-95.3056, 38.5263) (-95.3198, 38.4985) (-95.3339, 38.4707) (-95.3478, 38.4429) (-95.3616, 38.4151) (-95.3753, 38.3872) (-95.3888, 38.3593) (-95.4021, 38.3314) (-95.4153, 38.3035) (-95.4284, 38.2755) (-95.4413, 38.2476) (-95.4541, 38.2196) (-95.4667, 38.1916) (-95.4791, 38.1636) (-95.4914, 38.1355) (-95.5036, 38.1074) (-95.5155, 38.0794) (-95.5274, 38.0513) (-95.539, 38.0231) (-95.5505, 37.995) (-95.5619, 37.9668) (-95.5731, 37.9387) (-95.5841, 37.9105) (-95.5949, 37.8823) (-95.6056, 37.8541) (-95.6161, 37.8258) (-95.6265, 37.7976) (-95.6366, 37.7693) (-95.6466, 37.741) (-95.6565, 37.7128) (-95.6661, 37.6845) (-95.6756, 37.6561) (-95.6849, 37.6278) (-95.694, 37.5995) (-95.7029, 37.5711) (-95.7116, 37.5428) (-95.7202, 37.5144) (-95.7285, 37.486) (-95.7367, 37.4577) (-95.7446, 37.4293) (-95.7524, 37.4009) (-95.7599, 37.3725) (-95.7673, 37.344) (-95.7745, 37.3156) (-95.7814, 37.2872) (-95.7881, 37.2588) (-95.7945, 37.2303) (-95.8008, 37.2019) (-95.8068, 37.1735) (-95.8125, 37.145) (-95.8181, 37.1166) (-95.8234, 37.0881) (-95.8285, 37.0597) (-95.8334, 37.0313) (-95.8379, 37.0028) (-95.8421, 36.9744) (-95.8459, 36.946) (-95.8493, 36.9176) (-95.8524, 36.8891) (-95.8552, 36.8607) (-95.8579, 36.8324) (-95.8603, 36.804) (-95.8625, 36.7756) (-95.8642, 36.7473) (-95.8651, 36.719) (-95.8649, 36.6964) (-95.8642, 36.6794) (-95.8635, 36.6682) (-95.863, 36.6625) knots -1 -1 -1 -1 -1 -1 -0.98571429 -0.97142857 -0.95714286 -0.94285714 -0.92857143 -0.91428571 -0.9 -0.88571429 -0.87142857 -0.85714286 -0.84285714 -0.82857143 -0.81428571 -0.8 -0.78571429 -0.77142857 -0.75714286 -0.74285714 -0.72857143 -0.71428571 -0.7 -0.68571429 -0.67142857 -0.65714286 -0.64285714 -0.62857143 -0.61428571 -0.6 -0.58571429 -0.57142857 -0.55714286 -0.54285714 -0.52857143 -0.51428571 -0.5 -0.48571429 -0.47142857 -0.45714286 -0.44285714 -0.42857143 -0.41428571 -0.4 -0.38571429 -0.37142857 -0.35714286 -0.34285714 -0.32857143 -0.31428571 -0.3 -0.28571429 -0.27142857 -0.25714286 -0.24285714 -0.22857143 -0.21428571 -0.2 -0.18571429 -0.17142857 -0.15714286 -0.14285714 -0.12857143 -0.11428571 -0.1 -0.08571429 -0.07142857 -0.05714286 -0.04285714 -0.02857143 -0.01428571 0 0 0 0 0 0
  line L37 (-95.863, 36.6625) -> (-95.8246, 36.1768)
  arc A75 (-95.9154, 36.0693) -> (-95.8246, 36.1768) centre (-95.9242, 36.1689) ccw
  arc A76 (-95.9154, 36.0693) -> (-96.9298, 35.9358) centre (-94.8448, 24.0176) ccw
  arc A77 (-97.0454, 36.0161) -> (-96.9298, 35.9358) centre (-96.947, 36.0343) ccw
  line L38 (-97.0454, 36.0161) -> (-97.1339, 36.4952)
  spline S38 degree 5 poles (-97.1339, 36.4952) (-97.135, 36.5008) (-97.1371, 36.5119) (-97.1408, 36.5284) (-97.1465, 36.5503) (-97.1547, 36.5774) (-97.1637, 36.6043) (-97.1731, 36.6311) (-97.1829, 36.6579) (-97.1928, 36.6847) (-97.2029, 36.7113) (-97.2132, 36.738) (-97.2238, 36.7646) (-97.2349, 36.791) (-97.2463, 36.8174) (-97.258, 36.8437) (-97.27, 36.8699) (-97.2823, 36.8961) (-97.2949, 36.9222) (-97.3076, 36.9482) (-97.3205, 36.9742) (-97.3337, 37.0001) (-97.347, 37.0259) (-97.3606, 37.0517) (-97.3745, 37.0775) (-97.3885, 37.1031) (-97.4028, 37.1287) (-97.4172, 37.1543) (-97.4319, 37.1797) (-97.4467, 37.2052) (-97.4618, 37.2305) (-97.477, 37.2558) (-97.4924, 37.2811) (-97.508, 37.3063) (-97.5238, 37.3314) (-97.5397, 37.3565) (-97.5558, 37.3815) (-97.5722, 37.4065) (-97.5886, 37.4314) (-97.6053, 37.4562) (-97.6221, 37.481) (-97.6391, 37.5057) (-97.6562, 37.5304) (-97.6735, 37.555) (-97.691, 37.5795) (-97.7086, 37.604) (-97.7264, 37.6284) (-97.7443, 37.6528) (-97.7624, 37.6771) (-97.7806, 37.7014) (-97.799, 37.7256) (-97.8176, 37.7497) (-97.8363, 37.7738) (-97.8551, 37.7979) (-97.8741, 37.8218) (-97.8932, 37.8457) (-97.9125, 37.8696) (-97.9319, 37.8934) (-97.9515, 37.9171) (-97.9712, 37.9408) (-97.9911, 37.9644) (-98.011, 37.9879) (-98.0312, 38.0114) (-98.0514, 38.0349) (-98.0718, 38.0583) (-98.0924, 38.0816) (-98.113, 38.1048) (-98.1338, 38.128) (-98.1547, 38.1512) (-98.1758, 38.1742) (-98.197, 38.1972) (-98.2141, 38.2156) (-98.2269, 38.2294) (-98.2355, 38.2385) (-98.2398, 38.2431) knots 0 0 0 0 0 0 0.01428571 0.02857143 0.04285714 0.05714286 0.07142857 0.08571429 0.1 0.11428571 0.12857143 0.14285714 0.15714286 0.17142857 0.18571429 0.2 0.21428571 0.22857143 0.24285714 0.25714286 0.27142857 0.28571429 0.3 0.31428571 0.32857143 0.34285714 0.35714286 0.37142857 0.38571429 0.4 0.41428571 0.42857143 0.44285714 0.45714286 0.47142857 0.48571429 0.5 0.51428571 0.52857143 0.54285714 0.55714286 0.57142857 0.58571429 0.6 0.61428571 0.62857143 0.64285714 0.65714286 0.67142857 0.68571429 0.7 0.71428571 0.72857143 0.74285714 0.75714286 0.77142857 0.78571429 0.8 0.81428571 0.82857143 0.84285714 0.85714286 0.87142857 0.88571429 0.9 0.91428571 0.92857143 0.94285714 0.95714286 0.97142857 0.98571429 1 1 1 1 1 1
  arc A78 (-98.2398, 38.2431) -> (-99.0173, 38.0348) centre (-94.8448, 24.0176) ccw